Autodesk Fusion 360 part; units mm, degrees
(part 8 of 13)
  line L6244 (91.1132, -94.8176) -> (91.0017, -94.7608)
  line L6245 (101.955, -92.2213) -> (101.958, -92.1993)
  line L6246 (101.992, -92.133) -> (103.433, -90.6912)
  line L6247 (91.5604, -94.6723) -> (91.4719, -94.7608)
  line L6248 (103.086, -102.087) -> (103.021, -102.044)
  line L6249 (91.2368, -94.8372) -> (91.1132, -94.8176)
  line L6250 (103.457, -90.6736) -> (103.462, -90.6697)
  line L6251 (97.4257, -99.5716) -> (97.423, -99.5724)
  line L6252 (104.742, -90.9046) -> (103.574, -90.9046)
  line L6253 (105.254, -91.2108) -> (105.131, -91.2304)
  line L6254 (91.621, -94.5368) -> (91.6172, -94.5608)
  line L6255 (95.3324, -97.3037) -> (95.3333, -97.2973)
  line L6256 (95.7636, -96.8501) -> (95.7667, -96.8466)
  line L6257 (95.1296, -98.3423) -> (95.2181, -98.2538)
  line L6258 (95.6883, -98.2538) -> (95.7768, -98.3423)
  line L6259 (101.373, -94.0806) -> (101.373, -91.8718)
  line L6260 (103.434, -89.7635) -> (103.437, -89.76)
  line L6261 (95.2181, -98.901) -> (95.1296, -98.8125)
  line L6262 (95.8342, -96.8268) -> (96.127, -96.8268)
  line L6263 (108.504, -89.3456) -> (108.628, -89.4409)
  line L6264 (101.378, -91.8427) -> (101.379, -91.8363)
  line L6265 (95.2181, -98.2538) -> (95.3282, -98.1977)
  line L6266 (103.505, -89.7402) -> (107.62, -89.7402)
  line L6267 (107.684, -89.5652) -> (107.78, -89.4409)
  line L6268 (108.049, -89.2856) -> (108.204, -89.2652)
  line L6269 (95.7768, -98.3423) -> (95.8336, -98.4538)
  line L6270 (95.35, -97.2714) -> (95.3648, -97.2444)
  line L6271 (98.6272, -96.8268) -> (101.373, -94.0806)
  line L6272 (95.7694, -96.8458) -> (95.7746, -96.8419)
  line L6273 (95.8336, -98.4538) -> (95.8532, -98.5774)
  line L6274 (103.417, -89.7768) -> (103.434, -89.7635)
  line L6275 (105.131, -90.4304) -> (105.254, -90.45)
  line L6276 (96.127, -96.5818) -> (98.527, -96.5818)
  line L6277 (95.4532, -98.9774) -> (95.3296, -98.9578)
  line L6278 (105.007, -90.45) -> (105.131, -90.4304)
  line L6279 (95.7768, -98.8125) -> (95.6883, -98.901)
  line L6280 (108.204, -89.2652) -> (108.359, -89.2856)
  line L6281 (95.3311, -97.3062) -> (95.3324, -97.3037)
  line L6282 (101.373, -91.8718) -> (101.377, -91.8498)
  line L6283 (91.0017, -94.7608) -> (90.9132, -94.6723)
  line L6284 (92.1268, -99.3414) -> (97.3064, -99.3414)
  line L6285 (101.41, -91.7834) -> (103.417, -89.7768)
  line L6286 (95.6883, -98.901) -> (95.5768, -98.9578)
  line L6287 (95.0728, -98.4538) -> (95.1296, -98.3423)
  line L6288 (95.7458, -96.8634) -> (95.7636, -96.8501)
  line L6289 (95.3296, -98.9578) -> (95.2181, -98.901)
  line L6290 (95.3282, -97.3328) -> (95.3314, -97.3108)
  line L6291 (95.3648, -97.2444) -> (95.7458, -96.8634)
  line L6292 (95.5768, -98.9578) -> (95.4532, -98.9774)
  line L6293 (95.0532, -98.5774) -> (95.0728, -98.4538)
  line L6294 (107.904, -89.3456) -> (108.049, -89.2856)
  line L6295 (107.62, -89.7402) -> (107.624, -89.7099)
  line L6296 (103.475, -89.7489) -> (103.505, -89.7402)
  line L6297 (108.359, -89.2856) -> (108.504, -89.3456)
  line L6298 (107.624, -89.7099) -> (107.684, -89.5652)
  line L6299 (96.127, -96.8268) -> (96.127, -96.5818)
  line L6300 (101.377, -91.8498) -> (101.376, -91.8452)
  line L6301 (95.3333, -97.2973) -> (95.35, -97.2714)
  line L6302 (103.462, -90.6697) -> (103.492, -90.6633)
  line L6303 (95.8336, -98.701) -> (95.7768, -98.8125)
  line L6304 (103.445, -89.7553) -> (103.475, -89.7489)
  line L6305 (91.6172, -94.5608) -> (91.5604, -94.6723)
  line L6306 (95.1296, -98.8125) -> (95.0728, -98.701)
  line L6307 (98.527, -96.5818) -> (98.527, -96.8268)
  line L6308 (95.0728, -98.701) -> (95.0532, -98.5774)
  line L6309 (101.395, -91.8104) -> (101.41, -91.7834)
  line L6310 (103.437, -89.76) -> (103.44, -89.7592)
  line L6311 (95.8047, -96.8355) -> (95.8342, -96.8268)
  line L6312 (95.5782, -98.1977) -> (95.6883, -98.2538)
  line L6313 (95.3282, -98.1977) -> (95.3282, -97.3328)
  line L6314 (95.3314, -97.3108) -> (95.3311, -97.3062)
  line L6315 (101.379, -91.8363) -> (101.395, -91.8104)
  line L6316 (103.44, -89.7592) -> (103.445, -89.7553)
  line L6317 (95.7667, -96.8466) -> (95.7694, -96.8458)
  line L6318 (95.8532, -98.5774) -> (95.8336, -98.701)
  line L6319 (108.628, -89.4409) -> (108.724, -89.5652)
  line L6320 (122.123, -94.9134) -> (122, -94.8938)
  line L6321 (122.834, -95.4258) -> (122.812, -95.4226)
  line L6322 (121.743, -94.3898) -> (121.8, -94.2783)
  line L6323 (124.528, -95.406) -> (124.525, -95.4068)
  line L6324 (108.724, -90.1652) -> (108.628, -90.2895)
  line L6325 (98.7465, -97.057) -> (98.7438, -97.0578)
  line L6326 (122.773, -95.404) -> (122.746, -95.3892)
  line L6327 (101.619, -94.1615) -> (101.618, -94.1679)
  line L6328 (98.7496, -97.0535) -> (98.7465, -97.057)
  line L6329 (107.78, -90.2895) -> (107.684, -90.1652)
  line L6330 (98.527, -97.0768) -> (98.527, -97.3218)
  line L6331 (108.204, -90.4652) -> (108.049, -90.4448)
  line L6332 (96.127, -97.3218) -> (96.127, -97.0768)
  line L6333 (124.531, -95.4025) -> (124.528, -95.406)
  line L6334 (101.602, -94.1938) -> (101.587, -94.2208)
  line L6335 (95.7746, -96.8419) -> (95.8047, -96.8355)
  line L6336 (98.7085, -97.0681) -> (98.679, -97.0768)
  line L6337 (98.527, -97.3218) -> (96.127, -97.3218)
  line L6338 (101.587, -94.2208) -> (98.7674, -97.0402)
  line L6339 (124.52, -95.4107) -> (124.49, -95.4171)
  line L6340 (121.8, -94.2783) -> (121.888, -94.1898)
  line L6341 (121.743, -94.637) -> (121.723, -94.5134)
  line L6342 (107.624, -90.0205) -> (107.62, -89.9902)
  line L6343 (108.504, -90.3848) -> (108.359, -90.4448)
  line L6344 (95.5782, -97.3846) -> (95.5782, -98.1977)
  line L6345 (98.7438, -97.0578) -> (98.7386, -97.0617)
  line L6346 (108.784, -89.7099) -> (108.804, -89.8652)
  line L6347 (122.808, -95.4229) -> (122.805, -95.4216)
  line L6348 (101.621, -94.159) -> (101.619, -94.1615)
  line L6349 (98.679, -97.0768) -> (98.527, -97.0768)
  line L6350 (122.247, -94.8938) -> (122.123, -94.9134)
  line L6351 (98.527, -96.8268) -> (98.6272, -96.8268)
  line L6352 (121.888, -94.837) -> (121.8, -94.7485)
  line L6353 (107.78, -89.4409) -> (107.904, -89.3456)
  line L6354 (103.557, -89.9902) -> (101.623, -91.9236)
  line L6355 (101.623, -94.1324) -> (101.62, -94.1544)
  line L6356 (124.49, -95.4171) -> (124.46, -95.4258)
  line L6357 (122.746, -95.3892) -> (122.249, -94.8925)
  line L6358 (108.724, -89.5652) -> (108.784, -89.7099)
  line L6359 (122, -94.8938) -> (121.888, -94.837)
  line L6360 (121.8, -94.7485) -> (121.743, -94.637)
  line L6361 (108.804, -89.8652) -> (108.784, -90.0205)
  line L6362 (108.049, -90.4448) -> (107.904, -90.3848)
  line L6363 (101.376, -91.8452) -> (101.378, -91.8427)
  line L6364 (122.812, -95.4226) -> (122.808, -95.4229)
  line L6365 (122.249, -94.8925) -> (122.247, -94.8938)
  line L6366 (108.784, -90.0205) -> (108.724, -90.1652)
  line L6367 (101.62, -94.1544) -> (101.621, -94.159)
  line L6368 (107.684, -90.1652) -> (107.624, -90.0205)
  line L6369 (95.886, -97.0768) -> (95.5782, -97.3846)
  line L6370 (124.46, -95.4258) -> (122.834, -95.4258)
  line L6371 (107.904, -90.3848) -> (107.78, -90.2895)
  line L6372 (107.62, -89.9902) -> (103.557, -89.9902)
  line L6373 (108.359, -90.4448) -> (108.204, -90.4652)
  line L6374 (122.799, -95.4207) -> (122.773, -95.404)
  line L6375 (124.525, -95.4068) -> (124.52, -95.4107)
  line L6376 (98.7674, -97.0402) -> (98.7496, -97.0535)
  line L6377 (98.7386, -97.0617) -> (98.7085, -97.0681)
  line L6378 (101.618, -94.1679) -> (101.602, -94.1938)
  line L6379 (101.623, -91.9236) -> (101.623, -94.1324)
  line L6380 (108.628, -90.2895) -> (108.504, -90.3848)
  line L6381 (122.805, -95.4216) -> (122.799, -95.4207)
  line L6382 (121.723, -94.5134) -> (121.743, -94.3898)
  line L6383 (110.4, -92.9846) -> (110.305, -93.1089)
  line L6384 (122.504, -94.3898) -> (122.523, -94.5134)
  line L6385 (125.757, -92.0506) -> (124.484, -90.7776)
  line L6386 (113.296, -90.9442) -> (112.763, -91.4776)
  line L6387 (124.85, -94.7441) -> (124.874, -94.733)
  line L6388 (124.903, -94.7318) -> (125.692, -93.9424)
  line L6389 (122.447, -94.2783) -> (122.504, -94.3898)
  line L6390 (110.48, -92.6846) -> (110.46, -92.8399)
  line L6391 (124.778, -94.8048) -> (124.796, -94.7846)
  line L6392 (104.749, -96.9261) -> (104.816, -97.0341)
  line L6393 (122.451, -94.7405) -> (122.886, -95.1758)
  line L6394 (112.734, -91.4991) -> (112.704, -91.5055)
  line L6395 (121.888, -94.1898) -> (122, -94.133)
  line L6396 (109.297, -92.8096) -> (108.865, -92.8096)
  line L6397 (110.46, -92.8399) -> (110.4, -92.9846)
  line L6398 (124.408, -95.1758) -> (124.499, -95.0854)
  line L6399 (113.296, -90.9442) -> (113.296, -90.9442)
  line L6400 (113.463, -90.7776) -> (113.296, -90.9442)
  line L6401 (125.757, -93.8774) -> (125.757, -92.0506)
  line L6402 (125.692, -93.9424) -> (125.757, -93.8774)
  line L6403 (124.874, -94.733) -> (124.883, -94.7343)
  line L6404 (109.456, -93.1089) -> (109.361, -92.9846)
  line L6405 (104.715, -97.8403) -> (104.593, -97.9556)
  line L6406 (124.824, -94.7516) -> (124.85, -94.7441)
  line L6407 (110.4, -92.3846) -> (110.46, -92.5293)
  line L6408 (109.301, -92.8399) -> (109.297, -92.8096)
  line L6409 (104.89, -97.3791) -> (104.866, -97.5447)
  line L6410 (122.358, -94.1898) -> (122.447, -94.2783)
  line L6411 (112.742, -91.4944) -> (112.739, -91.4952)
  line L6412 (122.123, -94.1134) -> (122.247, -94.133)
  line L6413 (109.361, -92.9846) -> (109.301, -92.8399)
  line L6414 (104.866, -97.5447) -> (104.807, -97.701)
  line L6415 (110.305, -93.1089) -> (110.18, -93.2042)
  line L6416 (112.745, -91.4909) -> (112.742, -91.4944)
  line L6417 (104.807, -97.701) -> (104.715, -97.8403)
  line L6418 (124.892, -94.7318) -> (124.903, -94.7318)
  line L6419 (122.523, -94.5134) -> (122.504, -94.637)
  line L6420 (104.593, -97.9556) -> (104.45, -98.0412)
  line L6421 (124.81, -94.7622) -> (124.818, -94.7584)
  line L6422 (124.484, -90.7776) -> (113.463, -90.7776)
  line L6423 (124.796, -94.7846) -> (124.81, -94.7622)
  line L6424 (124.883, -94.7343) -> (124.892, -94.7318)
  line L6425 (104.816, -97.0341) -> (104.871, -97.192)
  line L6426 (124.778, -94.8061) -> (124.778, -94.8048)
  line L6427 (104.45, -98.0412) -> (104.291, -98.0929)
  line L6428 (112.704, -91.5055) -> (112.674, -91.5142)
  line L6429 (122, -94.133) -> (122.123, -94.1134)
  line L6430 (96.127, -97.0768) -> (95.886, -97.0768)
  line L6431 (112.763, -91.4776) -> (112.745, -91.4909)
  line L6432 (125.692, -93.9424) -> (125.692, -93.9424)
  line L6433 (108.865, -92.8096) -> (104.749, -96.9261)
  line L6434 (124.499, -95.0854) -> (124.778, -94.8061)
  line L6435 (110.18, -93.2042) -> (110.036, -93.2642)
  line L6436 (111.228, -91.5142) -> (110.381, -92.3604)
  line L6437 (109.725, -93.2642) -> (109.58, -93.2042)
  line L6438 (110.381, -92.3604) -> (110.4, -92.3846)
  line L6439 (112.739, -91.4952) -> (112.734, -91.4991)
  line L6440 (122.886, -95.1758) -> (124.408, -95.1758)
  line L6441 (112.674, -91.5142) -> (111.228, -91.5142)
  line L6442 (110.46, -92.5293) -> (110.48, -92.6846)
  line L6443 (124.818, -94.7584) -> (124.824, -94.7516)
  line L6444 (122.504, -94.637) -> (122.451, -94.7405)
  line L6445 (122.247, -94.133) -> (122.358, -94.1898)
  line L6446 (109.58, -93.2042) -> (109.456, -93.1089)
  line L6447 (104.311, -96.628) -> (104.469, -96.6841)
  line L6448 (109.725, -92.105) -> (109.88, -92.0846)
  line L6449 (103.678, -96.7672) -> (103.821, -96.6796)
  line L6450 (103.468, -97.0247) -> (103.559, -96.8842)
  line L6451 (111.116, -91.2793) -> (111.146, -91.2729)
  line L6452 (108.746, -92.5794) -> (108.749, -92.5786)
  line L6453 (103.406, -97.5141) -> (103.39, -97.3477)
  line L6454 (108.749, -92.5786) -> (108.754, -92.5747)
  line L6455 (109.297, -92.5596) -> (109.301, -92.5293)
  line L6456 (104.572, -96.7495) -> (108.725, -92.5962)
  line L6457 (113.343, -90.5474) -> (113.346, -90.5466)
  line L6458 (113.381, -90.5363) -> (113.411, -90.5276)
  line L6459 (124.536, -90.5276) -> (124.558, -90.5308)
  line L6460 (104.124, -98.108) -> (103.959, -98.0859)
  line L6461 (104.145, -96.6082) -> (104.311, -96.628)
  line L6462 (104.871, -97.192) -> (104.89, -97.3582)
  line L6463 (110.205, -92.1836) -> (111.087, -91.3008)
  line L6464 (124.625, -90.5642) -> (125.971, -91.9104)
  line L6465 (109.361, -92.3846) -> (109.456, -92.2603)
  line L6466 (113.323, -90.5642) -> (113.34, -90.5509)
  line L6467 (124.558, -90.5308) -> (124.563, -90.5305)
  line L6468 (109.88, -92.0846) -> (110.036, -92.105)
  line L6469 (103.959, -98.0859) -> (103.802, -98.0276)
  line L6470 (111.146, -91.2729) -> (111.176, -91.2642)
  line L6471 (113.351, -90.5427) -> (113.381, -90.5363)
  line L6472 (103.459, -97.6728) -> (103.406, -97.5141)
  line L6473 (103.411, -97.1818) -> (103.468, -97.0247)
  line L6474 (109.58, -92.165) -> (109.725, -92.105)
  line L6475 (113.34, -90.5509) -> (113.343, -90.5474)
  line L6476 (104.469, -96.6841) -> (104.572, -96.7495)
  line L6477 (104.291, -98.0929) -> (104.124, -98.108)
  line L6478 (110.036, -93.2642) -> (109.88, -93.2846)
  line L6479 (108.725, -92.5962) -> (108.743, -92.5829)
  line L6480 (108.743, -92.5829) -> (108.746, -92.5794)
  line L6481 (109.456, -92.2603) -> (109.58, -92.165)
  line L6482 (103.559, -96.8842) -> (103.678, -96.7672)
  line L6483 (103.39, -97.3477) -> (103.411, -97.1818)
  line L6484 (125.988, -91.9313) -> (125.988, -91.934)
  line L6485 (108.754, -92.5747) -> (108.784, -92.5683)
  line L6486 (108.814, -92.5596) -> (109.297, -92.5596)
  line L6487 (111.087, -91.3008) -> (111.105, -91.2875)
  line L6488 (125.984, -91.9282) -> (125.988, -91.9313)
  line L6489 (103.979, -96.6257) -> (104.145, -96.6082)
  line L6490 (103.662, -97.9361) -> (103.546, -97.8158)
  line L6491 (103.802, -98.0276) -> (103.662, -97.9361)
  line L6492 (113.346, -90.5466) -> (113.351, -90.5427)
  line L6493 (109.88, -93.2846) -> (109.725, -93.2642)
  line L6494 (103.821, -96.6796) -> (103.979, -96.6257)
  line L6495 (124.598, -90.5494) -> (124.625, -90.5642)
  line L6496 (113.119, -90.7674) -> (113.323, -90.5642)
  line L6497 (125.988, -91.934) -> (125.992, -91.9392)
  line L6498 (111.111, -91.2832) -> (111.116, -91.2793)
  line L6499 (124.565, -90.5318) -> (124.572, -90.5327)
  line L6500 (111.176, -91.2642) -> (112.623, -91.2642)
  line L6501 (110.036, -92.105) -> (110.18, -92.165)
  line L6502 (125.971, -91.9104) -> (125.984, -91.9282)
  line L6503 (124.563, -90.5305) -> (124.565, -90.5318)
  line L6504 (104.89, -97.3582) -> (104.89, -97.3791)
  line L6505 (103.546, -97.8158) -> (103.459, -97.6728)
  line L6506 (124.572, -90.5327) -> (124.598, -90.5494)
  line L6507 (112.623, -91.2642) -> (113.119, -90.7674)
  line L6508 (109.301, -92.5293) -> (109.361, -92.3846)
  line L6509 (108.784, -92.5683) -> (108.814, -92.5596)
  line L6510 (113.411, -90.5276) -> (124.536, -90.5276)
  line L6511 (111.266, -90.1652) -> (111.206, -90.0205)
  line L6512 (125.971, -94.0176) -> (125.869, -94.1192)
  line L6513 (125.022, -94.962) -> (125.02, -94.9628)
  line L6514 (125.869, -94.1192) -> (125.869, -94.1192)
  line L6515 (111.266, -89.5652) -> (111.284, -89.541)
  line L6516 (111.941, -89.2856) -> (112.085, -89.3456)
  line L6517 (112.365, -89.7099) -> (112.385, -89.8652)
  line L6518 (112.085, -90.3848) -> (111.941, -90.4448)
  line L6519 (111.108, -91.284) -> (111.111, -91.2832)
  line L6520 (113.119, -90.7674) -> (113.119, -90.7674)
  line L6521 (110.18, -92.165) -> (110.205, -92.1836)
  line L6522 (125.999, -91.9693) -> (126.007, -91.9988)
  line L6523 (125.992, -91.9392) -> (125.999, -91.9693)
  line L6524 (125.869, -94.1192) -> (125.043, -94.9452)
  line L6525 (111.206, -90.0205) -> (111.185, -89.8652)
  line L6526 (111.284, -89.541) -> (110.692, -88.9488)
  line L6527 (110.78, -88.7039) -> (110.805, -88.7206)
  line L6528 (110.773, -88.703) -> (110.78, -88.7039)
  line L6529 (94.6272, -97.0402) -> (94.627, -97.0403)
  line L6530 (111.485, -90.3848) -> (111.361, -90.2895)
  line L6531 (95.8017, -95.8443) -> (95.785, -95.8702)
  line L6532 (111.361, -90.2895) -> (111.266, -90.1652)
  line L6533 (112.085, -89.3456) -> (112.21, -89.4409)
  line L6534 (125.025, -94.9585) -> (125.022, -94.962)
  line L6535 (110.692, -88.9488) -> (97.7656, -88.9488)
  line L6536 (95.8068, -95.8088) -> (95.8036, -95.8308)
  line L6537 (111.785, -90.4652) -> (111.63, -90.4448)
  line L6538 (110.832, -88.7354) -> (111.461, -89.3642)
  line L6539 (125.043, -94.9452) -> (125.025, -94.9585)
  line L6540 (111.485, -89.3456) -> (111.63, -89.2856)
  line L6541 (124.984, -94.9731) -> (124.956, -94.9814)
  line L6542 (124.956, -94.9814) -> (124.548, -95.3892)
  line L6543 (125.986, -93.9906) -> (125.971, -94.0176)
  line L6544 (126.003, -93.9583) -> (126.002, -93.9647)
  line L6545 (111.461, -89.3642) -> (111.485, -89.3456)
  line L6546 (126.002, -93.9647) -> (125.986, -93.9906)
  line L6547 (124.548, -95.3892) -> (124.531, -95.4025)
  line L6548 (111.63, -89.2856) -> (111.785, -89.2652)
  line L6549 (126.005, -93.9558) -> (126.003, -93.9583)
  line L6550 (112.305, -89.5652) -> (112.365, -89.7099)
  line L6551 (110.805, -88.7206) -> (110.832, -88.7354)
  line L6552 (111.185, -89.8652) -> (111.206, -89.7099)
  line L6553 (112.385, -89.8652) -> (112.365, -90.0205)
  line L6554 (97.7656, -88.9488) -> (95.8068, -90.9076)
  line L6555 (125.014, -94.9667) -> (124.984, -94.9731)
  line L6556 (111.63, -90.4448) -> (111.485, -90.3848)
  line L6557 (125.02, -94.9628) -> (125.014, -94.9667)
  line L6558 (126.004, -93.9512) -> (126.005, -93.9558)
  line L6559 (111.785, -89.2652) -> (111.941, -89.2856)
  line L6560 (126.007, -91.9988) -> (126.007, -93.9292)
  line L6561 (110.766, -88.702) -> (110.771, -88.7017)
  line L6562 (110.771, -88.7017) -> (110.773, -88.703)
  line L6563 (111.105, -91.2875) -> (111.108, -91.284)
  line L6564 (95.8026, -95.8379) -> (95.8017, -95.8443)
  line L6565 (95.8039, -95.8354) -> (95.8026, -95.8379)
  line L6566 (111.941, -90.4448) -> (111.785, -90.4652)
  line L6567 (126.007, -93.9292) -> (126.004, -93.9512)
  line L6568 (112.21, -90.2895) -> (112.085, -90.3848)
  line L6569 (112.21, -89.4409) -> (112.305, -89.5652)
  line L6570 (95.8068, -90.9076) -> (95.8068, -95.8088)
  line L6571 (112.305, -90.1652) -> (112.21, -90.2895)
  line L6572 (95.8036, -95.8308) -> (95.8039, -95.8354)
  line L6573 (111.206, -89.7099) -> (111.266, -89.5652)
  line L6574 (95.785, -95.8702) -> (95.7702, -95.8972)
  line L6575 (118.156, -93.4328) -> (118.011, -93.4928)
  line L6576 (95.5786, -90.7944) -> (95.5934, -90.7674)
  line L6577 (91.6172, -97.2346) -> (91.6368, -97.3582)
  line L6578 (110.744, -88.6988) -> (110.766, -88.702)
  line L6579 (90.8564, -97.4818) -> (90.8368, -97.3582)
  line L6580 (118.436, -93.0685) -> (118.376, -93.2132)
  line L6581 (95.5568, -95.757) -> (95.5568, -90.8558)
  line L6582 (97.649, -88.7178) -> (97.6542, -88.7139)
  line L6583 (97.6843, -88.7075) -> (97.7138, -88.6988)
  line L6584 (118.376, -93.2132) -> (118.28, -93.3375)
  line L6585 (91.5604, -97.5933) -> (91.4719, -97.6818)
  line L6586 (118.156, -92.3936) -> (118.28, -92.4889)
  line L6587 (92.227, -96.5818) -> (94.627, -96.5818)
  line L6588 (94.627, -97.0403) -> (94.627, -97.3218)
  line L6589 (90.8368, -97.3582) -> (90.8564, -97.2346)
  line L6590 (118.436, -92.7579) -> (118.456, -92.9132)
  line L6591 (91.695, -97.0768) -> (91.5902, -97.1816)
  line L6592 (91.5784, -96.8458) -> (91.5836, -96.8419)
  line L6593 (112.365, -90.0205) -> (112.305, -90.1652)
  line L6594 (91.3604, -97.7386) -> (91.2368, -97.7582)
  line L6595 (91.6172, -97.4818) -> (91.5604, -97.5933)
  line L6596 (91.0017, -97.0346) -> (91.1132, -96.9778)
  line L6597 (90.9132, -97.1231) -> (91.0017, -97.0346)
  line L6598 (91.1132, -97.7386) -> (91.0017, -97.6818)
  line L6599 (94.627, -97.3218) -> (92.227, -97.3218)
  line L6600 (91.4134, -97.0048) -> (91.5548, -96.8634)
  line L6601 (90.8564, -97.2346) -> (90.9132, -97.1231)
  line L6602 (95.7702, -95.8972) -> (94.6272, -97.0402)
  line L6603 (94.627, -96.6868) -> (95.5568, -95.757)
  line L6604 (91.1132, -96.9778) -> (91.2368, -96.9582)
  line L6605 (92.227, -96.8268) -> (92.227, -96.5818)
  line L6606 (90.9132, -97.5933) -> (90.8564, -97.4818)
  line L6607 (97.6254, -88.7354) -> (97.6432, -88.7221)
  line L6608 (97.6463, -88.7186) -> (97.649, -88.7178)
  line L6609 (118.456, -92.9132) -> (118.436, -93.0685)
  line L6610 (97.6432, -88.7221) -> (97.6463, -88.7186)
  line L6611 (91.4719, -97.6818) -> (91.3604, -97.7386)
  line L6612 (91.2368, -96.9582) -> (91.3604, -96.9778)
  line L6613 (91.5757, -96.8466) -> (91.5784, -96.8458)
  line L6614 (95.56, -90.8338) -> (95.5597, -90.8292)
  line L6615 (118.28, -93.3375) -> (118.156, -93.4328)
  line L6616 (95.5934, -90.7674) -> (97.6254, -88.7354)
  line L6617 (95.5568, -90.8558) -> (95.56, -90.8338)
  line L6618 (91.6137, -96.8355) -> (91.6432, -96.8268)
  line L6619 (95.5619, -90.8203) -> (95.5786, -90.7944)
  line L6620 (91.5836, -96.8419) -> (91.6137, -96.8355)
  line L6621 (91.2368, -97.7582) -> (91.1132, -97.7386)
  line L6622 (91.0017, -97.6818) -> (90.9132, -97.5933)
  line L6623 (91.5548, -96.8634) -> (91.5726, -96.8501)
  line L6624 (91.6432, -96.8268) -> (92.227, -96.8268)
  line L6625 (92.227, -97.0768) -> (91.695, -97.0768)
  line L6626 (118.28, -92.4889) -> (118.376, -92.6132)
  line L6627 (91.6368, -97.3582) -> (91.6172, -97.4818)
  line L6628 (91.5726, -96.8501) -> (91.5757, -96.8466)
  line L6629 (91.5902, -97.1816) -> (91.6172, -97.2346)
  line L6630 (118.011, -92.3336) -> (118.156, -92.3936)
  line L6631 (118.376, -92.6132) -> (118.436, -92.7579)
  line L6632 (92.227, -97.3218) -> (92.227, -97.0768)
  line L6633 (95.5597, -90.8292) -> (95.561, -90.8267)
  line L6634 (97.6542, -88.7139) -> (97.6843, -88.7075)
  line L6635 (94.627, -96.5818) -> (94.627, -96.6868)
  line L6636 (97.7138, -88.6988) -> (110.744, -88.6988)
  line L6637 (91.3604, -96.9778) -> (91.4134, -97.0048)
  line L6638 (95.561, -90.8267) -> (95.5619, -90.8203)
  line L6639 (117.295, -93.6508) -> (117.295, -95.7843)
  line L6640 (117.295, -95.7843) -> (117.341, -95.7898)
  line L6641 (117.048, -93.5724) -> (117.049, -93.5699)
  line L6642 (117.837, -96.8628) -> (117.745, -97.0021)
  line L6643 (114.566, -92.3338) -> (114.626, -92.4785)
  line L6644 (117.082, -93.5106) -> (117.355, -93.2374)
  line L6645 (114.346, -93.1534) -> (114.201, -93.2134)
  line L6646 (117.624, -97.1174) -> (117.48, -97.203)
  line L6647 (117.701, -93.4928) -> (117.556, -93.4328)
  line L6648 (116.708, -95.929) -> (116.851, -95.8414)
  line L6649 (117.432, -92.4889) -> (117.556, -92.3936)
  line L6650 (114.646, -92.6338) -> (114.626, -92.7891)
  line L6651 (116.489, -96.8346) -> (116.437, -96.6759)
  line L6652 (114.201, -93.2134) -> (114.046, -93.2338)
  line L6653 (117.045, -93.599) -> (117.048, -93.577)
  line L6654 (117.048, -93.577) -> (117.048, -93.5724)
  line L6655 (117.92, -96.52) -> (117.92, -96.5409)
  line L6656 (117.321, -97.2547) -> (117.154, -97.2698)
  line L6657 (116.437, -96.6759) -> (116.42, -96.5095)
  line L6658 (116.692, -97.0979) -> (116.576, -96.9776)
  line L6659 (117.05, -93.5635) -> (117.067, -93.5376)
  line L6660 (117.276, -93.0685) -> (117.256, -92.9132)
  line L6661 (116.989, -97.2477) -> (116.832, -97.1894)
  line L6662 (114.47, -93.0581) -> (114.346, -93.1534)
  line L6663 (118.011, -93.4928) -> (117.856, -93.5132)
  line L6664 (117.856, -92.3132) -> (118.011, -92.3336)
  line L6665 (116.589, -96.046) -> (116.708, -95.929)
  line L6666 (117.902, -96.3538) -> (117.92, -96.52)
  line L6667 (116.576, -96.9776) -> (116.489, -96.8346)
  line L6668 (117.897, -96.7065) -> (117.837, -96.8628)
  line L6669 (114.566, -92.9338) -> (114.47, -93.0581)
  line L6670 (117.049, -93.5699) -> (117.05, -93.5635)
  line L6671 (117.532, -93.4142) -> (117.295, -93.6508)
  line L6672 (117.745, -97.0021) -> (117.624, -97.1174)
  line L6673 (117.48, -97.203) -> (117.321, -97.2547)
  line L6674 (117.154, -97.2698) -> (116.989, -97.2477)
  line L6675 (116.851, -95.8414) -> (117.009, -95.7875)
  line L6676 (117.256, -92.9132) -> (117.276, -92.7579)
  line L6677 (117.276, -92.7579) -> (117.336, -92.6132)
  line L6678 (114.346, -92.1142) -> (114.47, -92.2095)
  line L6679 (117.556, -93.4328) -> (117.532, -93.4142)
  line L6680 (117.758, -96.0541) -> (117.847, -96.1959)
  line L6681 (117.701, -92.3336) -> (117.856, -92.3132)
  line L6682 (114.626, -92.4785) -> (114.646, -92.6338)
  line L6683 (116.832, -97.1894) -> (116.692, -97.0979)
  line L6684 (116.498, -96.1865) -> (116.589, -96.046)
  line L6685 (117.045, -95.7837) -> (117.045, -93.599)
  line L6686 (116.42, -96.5095) -> (116.441, -96.3436)
  line L6687 (117.009, -95.7875) -> (117.045, -95.7837)
  line L6688 (117.92, -96.5409) -> (117.897, -96.7065)
  line L6689 (117.847, -96.1959) -> (117.902, -96.3538)
  line L6690 (117.336, -92.6132) -> (117.432, -92.4889)
  line L6691 (114.626, -92.7891) -> (114.566, -92.9338)
  line L6692 (114.47, -92.2095) -> (114.566, -92.3338)
  line L6693 (117.355, -93.2374) -> (117.336, -93.2132)
  line L6694 (117.556, -92.3936) -> (117.701, -92.3336)
  line L6695 (114.201, -92.0542) -> (114.346, -92.1142)
  line L6696 (117.64, -95.9355) -> (117.758, -96.0541)
  line L6697 (117.336, -93.2132) -> (117.276, -93.0685)
  line L6698 (117.341, -95.7898) -> (117.499, -95.8459)
  line L6699 (117.856, -93.5132) -> (117.701, -93.4928)
  line L6700 (117.499, -95.8459) -> (117.64, -95.9355)
  line L6701 (116.441, -96.3436) -> (116.498, -96.1865)
  line L6702 (117.067, -93.5376) -> (117.082, -93.5106)
  line L6703 (124.375, -94.6186) -> (124.372, -94.6194)
  line L6704 (113.746, -92.1142) -> (113.891, -92.0542)
  line L6705 (114.396, -96.8628) -> (114.303, -97.0021)
  line L6706 (113.879, -97.2547) -> (113.713, -97.2698)
  line L6707 (113.25, -97.0979) -> (113.134, -96.9776)
  line L6708 (124.344, -91.2098) -> (124.371, -91.2246)
  line L6709 (114.455, -96.7065) -> (114.396, -96.8628)
  line L6710 (124.372, -94.6194) -> (124.367, -94.6233)
  line L6711 (125.425, -92.2838) -> (125.429, -92.2869)
  line L6712 (125.449, -92.3544) -> (125.449, -93.4974)
  line L6713 (113.547, -97.2477) -> (113.39, -97.1894)
  line L6714 (125.433, -92.2948) -> (125.44, -92.3249)
  line L6715 (125.44, -92.3249) -> (125.449, -92.3544)
  line L6716 (125.445, -93.5194) -> (125.446, -93.524)
  line L6717 (112.979, -96.5095) -> (113, -96.3436)
  line L6718 (113.39, -97.1894) -> (113.25, -97.0979)
  line L6719 (124.367, -94.6233) -> (124.337, -94.6297)
  line L6720 (113.853, -93.1979) -> (113.853, -95.7843)
  line L6721 (113.147, -96.046) -> (113.267, -95.929)
  line L6722 (112.995, -96.6759) -> (112.979, -96.5095)
  line L6723 (125.446, -93.524) -> (125.444, -93.5265)
  line L6724 (125.412, -92.266) -> (125.425, -92.2838)
  line L6725 (113.048, -96.8346) -> (112.995, -96.6759)
  line L6726 (114.316, -96.0541) -> (114.405, -96.1959)
  line L6727 (114.057, -95.8459) -> (114.198, -95.9355)
  line L6728 (113.446, -92.6338) -> (113.466, -92.4785)
  line L6729 (113.466, -92.7891) -> (113.446, -92.6338)
  line L6730 (124.318, -91.1931) -> (124.344, -91.2098)
  line L6731 (124.311, -91.1922) -> (124.318, -91.1931)
  line L6732 (125.429, -92.2869) -> (125.43, -92.2896)
  line L6733 (114.478, -96.5409) -> (114.455, -96.7065)
  line L6734 (114.303, -97.0021) -> (114.182, -97.1174)
  line L6735 (113.9, -95.7898) -> (114.057, -95.8459)
  line L6736 (113.409, -95.8414) -> (113.567, -95.7875)
  line L6737 (113, -96.3436) -> (113.057, -96.1865)
  line L6738 (114.038, -97.203) -> (113.879, -97.2547)
  line L6739 (114.46, -96.3538) -> (114.478, -96.52)
  line L6740 (113.134, -96.9776) -> (113.048, -96.8346)
  line L6741 (113.891, -93.2134) -> (113.853, -93.1979)
  line L6742 (114.198, -95.9355) -> (114.316, -96.0541)
  line L6743 (114.405, -96.1959) -> (114.46, -96.3538)
  line L6744 (113.713, -97.2698) -> (113.547, -97.2477)
  line L6745 (125.449, -93.4974) -> (125.445, -93.5194)
  line L6746 (125.43, -92.2896) -> (125.433, -92.2948)
  line L6747 (124.396, -94.6018) -> (124.378, -94.6151)
  line L6748 (125.444, -93.5265) -> (125.443, -93.5329)
  line L6749 (114.182, -97.1174) -> (114.038, -97.203)
  line L6750 (113.526, -92.9338) -> (113.466, -92.7891)
  line L6751 (113.267, -95.929) -> (113.409, -95.8414)
  line L6752 (125.412, -93.5858) -> (124.396, -94.6018)
  line L6753 (113.603, -95.7837) -> (113.603, -93.0343)
  line L6754 (124.371, -91.2246) -> (125.412, -92.266)
  line L6755 (124.304, -91.1912) -> (124.309, -91.1909)
  line L6756 (113.567, -95.7875) -> (113.603, -95.7837)
  line L6757 (114.046, -92.0338) -> (114.201, -92.0542)
  line L6758 (125.427, -93.5588) -> (125.412, -93.5858)
  line L6759 (124.378, -94.6151) -> (124.375, -94.6186)
  line L6760 (113.853, -95.7843) -> (113.9, -95.7898)
  line L6761 (113.603, -93.0343) -> (113.526, -92.9338)
  line L6762 (113.057, -96.1865) -> (113.147, -96.046)
  line L6763 (113.891, -92.0542) -> (114.046, -92.0338)
  line L6764 (113.622, -92.2095) -> (113.746, -92.1142)
  line L6765 (114.046, -93.2338) -> (113.891, -93.2134)
  line L6766 (114.478, -96.52) -> (114.478, -96.5409)
  line L6767 (113.526, -92.3338) -> (113.622, -92.2095)
  line L6768 (124.23, -91.438) -> (113.488, -91.438)
  line L6769 (125.199, -93.4456) -> (125.199, -92.4062)
  line L6770 (112.559, -92.41) -> (112.619, -92.5547)
  line L6771 (123.578, -94.7485) -> (123.521, -94.637)
  line L6772 (125.443, -93.5329) -> (125.427, -93.5588)
  line L6773 (124.309, -91.1909) -> (124.311, -91.1922)
  line L6774 (125.199, -92.4062) -> (124.23, -91.438)
  line L6775 (112.54, -92.3858) -> (112.559, -92.41)
  line L6776 (112.639, -92.71) -> (112.619, -92.8653)
  line L6777 (112.619, -92.8653) -> (112.559, -93.01)
  line L6778 (113.466, -92.4785) -> (113.526, -92.3338)
  line L6779 (100.591, -89.5793) -> (100.679, -89.4908)
  line L6780 (98.9243, -91.977) -> (98.9216, -91.9778)
  line L6781 (112.468, -85.2378) -> (112.324, -85.1778)
  line L6782 (100.738, -90.1678) -> (98.9452, -91.9602)
  line L6783 (112.044, -84.8135) -> (112.024, -84.6582)
  line L6784 (90.7548, -91.97) -> (90.7352, -91.8464)
  line L6785 (91.0116, -91.466) -> (91.1352, -91.4464)
  line L6786 (101.185, -83.5831) -> (101.215, -83.5767)
  line L6787 (101.18, -83.587) -> (101.185, -83.5831)
  line L6788 (100.679, -89.4908) -> (100.791, -89.434)
  line L6789 (93.3062, -91.4813) -> (93.3071, -91.4749)
  line L6790 (100.791, -89.434) -> (100.914, -89.4144)
  line L6791 (113.048, -85.0825) -> (112.924, -85.1778)
  line L6792 (113.143, -84.9582) -> (113.048, -85.0825)
  line L6793 (98.8568, -91.9968) -> (98.527, -91.9968)
  line L6794 (111.658, -83.568) -> (111.68, -83.5712)
  line L6795 (113.224, -84.6582) -> (113.203, -84.8135)
  line L6796 (91.1352, -91.4464) -> (91.2588, -91.466)
  line L6797 (93.3238, -91.449) -> (93.3386, -91.422)
  line L6798 (91.4588, -91.6113) -> (91.5156, -91.7228)
  line L6799 (113.203, -84.5029) -> (113.224, -84.6582)
  line L6800 (93.6124, -91.5018) -> (94.627, -91.5018)
  line L6801 (113.048, -84.2339) -> (113.143, -84.3582)
  line L6802 (113.143, -84.3582) -> (113.203, -84.5029)
  line L6803 (90.7352, -91.8464) -> (90.7548, -91.7228)
  line L6804 (93.3386, -91.422) -> (101.156, -83.6046)
  line L6805 (112.123, -84.334) -> (111.607, -83.818)
  line L6806 (91.5194, -91.7468) -> (92.227, -91.7468)
  line L6807 (93.3052, -91.4884) -> (93.3049, -91.4838)
  line L6808 (90.9001, -92.17) -> (90.8116, -92.0815)
  line L6809 (91.0116, -92.2268) -> (90.9001, -92.17)
  line L6810 (111.607, -83.818) -> (101.296, -83.818)
  line L6811 (92.227, -91.7468) -> (92.227, -91.5018)
  line L6812 (101.177, -83.5878) -> (101.18, -83.587)
  line L6813 (90.9001, -91.5228) -> (91.0116, -91.466)
  line L6814 (93.3071, -91.4749) -> (93.3238, -91.449)
  line L6815 (94.627, -91.5018) -> (94.627, -92.2418)
  line L6816 (91.1352, -92.2464) -> (91.0116, -92.2268)
  line L6817 (112.044, -84.5029) -> (112.104, -84.3582)
  line L6818 (90.7548, -91.7228) -> (90.8116, -91.6113)
  line L6819 (101.238, -89.5793) -> (101.295, -89.6908)
  line L6820 (96.127, -91.5018) -> (98.527, -91.5018)
  line L6821 (90.8116, -91.6113) -> (90.9001, -91.5228)
  line L6822 (112.024, -84.6582) -> (112.044, -84.5029)
  line L6823 (90.8116, -92.0815) -> (90.7548, -91.97)
  line L6824 (113.203, -84.8135) -> (113.143, -84.9582)
  line L6825 (112.199, -85.0825) -> (112.104, -84.9582)
  line L6826 (112.624, -85.2582) -> (112.468, -85.2378)
  line L6827 (91.2588, -91.466) -> (91.3703, -91.5228)
  line L6828 (93.3032, -91.5018) -> (93.3052, -91.4884)
  line L6829 (101.174, -83.5913) -> (101.177, -83.5878)
  line L6830 (92.227, -91.5018) -> (93.3032, -91.5018)
  line L6831 (101.296, -83.818) -> (93.6124, -91.5018)
  line L6832 (112.779, -85.2378) -> (112.624, -85.2582)
  line L6833 (91.3703, -91.5228) -> (91.4588, -91.6113)
  line L6834 (101.156, -83.6046) -> (101.174, -83.5913)
  line L6835 (101.244, -83.568) -> (111.658, -83.568)
  line L6836 (93.3049, -91.4838) -> (93.3062, -91.4813)
  line L6837 (101.215, -83.5767) -> (101.244, -83.568)
  line L6838 (101.038, -89.434) -> (101.149, -89.4908)
  line L6839 (91.5156, -91.7228) -> (91.5194, -91.7468)
  line L6840 (100.534, -89.6908) -> (100.591, -89.5793)
  line L6841 (92.227, -92.2418) -> (92.227, -91.9968)
  line L6842 (98.527, -92.2418) -> (96.127, -92.2418)
  line L6843 (100.534, -89.938) -> (100.514, -89.8144)
  line L6844 (101.149, -90.138) -> (101.038, -90.1948)
  line L6845 (101.038, -90.1948) -> (100.914, -90.2144)
  line L6846 (98.9274, -91.9735) -> (98.9243, -91.977)
  line L6847 (100.561, -89.991) -> (100.534, -89.938)
  line L6848 (101.238, -90.0495) -> (101.149, -90.138)
  line L6849 (101.314, -89.8144) -> (101.295, -89.938)
  line L6850 (98.9164, -91.9817) -> (98.8863, -91.9881)
  line L6851 (98.527, -91.9968) -> (98.527, -92.2418)
  line L6852 (96.127, -92.2418) -> (96.127, -91.5018)
  line L6853 (100.514, -89.8144) -> (100.534, -89.6908)
  line L6854 (98.527, -91.7468) -> (98.805, -91.7468)
  line L6855 (98.527, -91.5018) -> (98.527, -91.7468)
  line L6856 (100.791, -90.1948) -> (100.738, -90.1678)
  line L6857 (100.914, -90.2144) -> (100.791, -90.1948)
  line L6858 (101.295, -89.938) -> (101.238, -90.0495)
  line L6859 (101.149, -89.4908) -> (101.238, -89.5793)
  line L6860 (129.766, -91.8672) -> (129.621, -91.8072)
  line L6861 (101.295, -89.6908) -> (101.314, -89.8144)
  line L6862 (129.921, -91.8876) -> (129.766, -91.8672)
  line L6863 (98.9216, -91.9778) -> (98.9164, -91.9817)
  line L6864 (98.9452, -91.9602) -> (98.9274, -91.9735)
  line L6865 (98.8863, -91.9881) -> (98.8568, -91.9968)
  line L6866 (98.805, -91.7468) -> (100.561, -89.991)
  line L6867 (130.076, -91.8672) -> (129.921, -91.8876)
  line L6868 (129.497, -91.7119) -> (129.401, -91.5876)
  line L6869 (129.401, -91.5876) -> (129.341, -91.4429)
  line L6870 (129.621, -90.768) -> (129.766, -90.708)
  line L6871 (135.943, -71.3229) -> (136.061, -71.4415)
  line L6872 (136.061, -71.4415) -> (136.15, -71.5833)
  line L6873 (129.341, -91.4429) -> (129.321, -91.2876)
  line L6874 (130.441, -90.9876) -> (130.501, -91.1323)
  line L6875 (130.221, -90.768) -> (130.345, -90.8633)
  line L6876 (130.521, -91.2876) -> (130.501, -91.4429)
  line L6877 (100.914, -89.4144) -> (101.038, -89.434)
  line L6878 (136.205, -71.7412) -> (136.223, -71.9074)
  line L6879 (136.15, -71.5833) -> (136.205, -71.7412)
  line L6880 (130.345, -90.8633) -> (130.441, -90.9876)
  line L6881 (136.223, -71.9074) -> (136.223, -71.9283)
  line L6882 (130.441, -91.5876) -> (130.345, -91.7119)
  line L6883 (130.345, -91.7119) -> (130.221, -91.8072)
  line L6884 (129.497, -90.8633) -> (129.621, -90.768)
  line L6885 (135.802, -71.2333) -> (135.943, -71.3229)
  line L6886 (130.501, -91.1323) -> (130.521, -91.2876)
  line L6887 (129.321, -91.2876) -> (129.341, -91.1323)
  line L6888 (129.921, -90.6876) -> (130.076, -90.708)
  line L6889 (129.766, -90.708) -> (129.921, -90.6876)
  line L6890 (129.621, -91.8072) -> (129.497, -91.7119)
  line L6891 (129.401, -90.9876) -> (129.497, -90.8633)
  line L6892 (136.223, -71.9283) -> (136.2, -72.0939)
  line L6893 (133.968, -83.4302) -> (133.974, -83.4603)
  line L6894 (133.983, -83.4898) -> (133.983, -90.5263)
  line L6895 (134.013, -90.5302) -> (134.158, -90.5902)
  line L6896 (133.974, -83.4603) -> (133.983, -83.4898)
  line L6897 (135.645, -71.1772) -> (135.802, -71.2333)
  line L6898 (134.158, -90.5902) -> (134.282, -90.6855)
  line L6899 (136.141, -72.2502) -> (136.048, -72.3895)
  line L6900 (130.501, -91.4429) -> (130.441, -91.5876)
  line L6901 (135.598, -81.6204) -> (135.595, -81.6424)
  line L6902 (130.076, -90.708) -> (130.221, -90.768)
  line L6903 (129.341, -91.1323) -> (129.401, -90.9876)
  line L6904 (130.221, -91.8072) -> (130.076, -91.8672)
  line L6905 (134.458, -91.1098) -> (134.438, -91.2651)
  line L6906 (135.595, -81.6424) -> (135.596, -81.647)
  line L6907 (134.282, -90.6855) -> (134.378, -90.8098)
  line L6908 (135.927, -72.5048) -> (135.783, -72.5904)
  line L6909 (135.593, -81.6559) -> (135.577, -81.6817)
  line L6910 (112.339, -92.1904) -> (112.364, -92.209)
  line L6911 (111.46, -92.5547) -> (111.52, -92.41)
  line L6912 (110.166, -94.4335) -> (110.167, -94.4271)
  line L6913 (111.739, -92.1904) -> (111.884, -92.1304)
  line L6914 (110.162, -95.7837) -> (110.162, -94.4626)
  line L6915 (110.184, -94.4012) -> (110.198, -94.3742)
  line L6916 (110.126, -95.7875) -> (110.162, -95.7837)
  line L6917 (112.364, -92.209) -> (113.348, -91.2246)
  line L6918 (113.436, -91.188) -> (124.282, -91.188)
  line L6919 (109.967, -95.8414) -> (110.126, -95.7875)
  line L6920 (110.165, -94.4406) -> (110.165, -94.436)
  line L6921 (111.884, -92.1304) -> (112.039, -92.11)
  line L6922 (113.377, -91.2031) -> (113.407, -91.1967)
  line L6923 (113.407, -91.1967) -> (113.436, -91.188)
  line L6924 (109.825, -95.929) -> (109.967, -95.8414)
  line L6925 (112.195, -92.1304) -> (112.339, -92.1904)
  line L6926 (113.366, -91.2113) -> (113.369, -91.2078)
  line L6927 (111.46, -92.8653) -> (111.439, -92.71)
  line L6928 (111.439, -92.71) -> (111.46, -92.5547)
  line L6929 (111.52, -93.01) -> (111.46, -92.8653)
  line L6930 (111.615, -92.2857) -> (111.739, -92.1904)
  line L6931 (110.198, -94.3742) -> (111.538, -93.0342)
  line L6932 (111.52, -92.41) -> (111.615, -92.2857)
  line L6933 (109.706, -96.046) -> (109.825, -95.929)
  line L6934 (113.369, -91.2078) -> (113.372, -91.207)
  line L6935 (111.538, -93.0342) -> (111.52, -93.01)
  line L6936 (110.165, -94.436) -> (110.166, -94.4335)
  line L6937 (110.162, -94.4626) -> (110.165, -94.4406)
  line L6938 (131.747, -96.9696) -> (131.347, -96.9696)
  line L6939 (132.355, -95.8354) -> (132.353, -95.8379)
  line L6940 (134.017, -96.8204) -> (134.002, -96.8969)
  line L6941 (132.353, -95.8379) -> (132.352, -95.8443)
  line L6942 (131.931, -96.8461) -> (131.888, -96.911)
  line L6943 (133.24, -96.1825) -> (133.276, -96.129)
  line L6944 (132.613, -94.9999) -> (132.556, -95.1114)
  line L6945 (132.556, -94.6412) -> (132.613, -94.7527)
  line L6946 (131.909, -95.1114) -> (131.852, -94.9999)
  line L6947 (133.817, -96.0704) -> (133.894, -96.0856)
  line L6948 (131.997, -95.1999) -> (131.909, -95.1114)
  line L6949 (132.556, -95.1114) -> (132.468, -95.1999)
  line L6950 (131.162, -96.1431) -> (131.205, -96.0782)
  line L6951 (131.888, -96.911) -> (131.823, -96.9544)
  line L6952 (133.276, -96.129) -> (133.341, -96.0856)
  line L6953 (134.017, -96.2704) -> (134.017, -96.8204)
  line L6954 (124.282, -91.188) -> (124.304, -91.1912)
  line L6955 (132.109, -94.4959) -> (132.232, -94.4763)
  line L6956 (131.852, -94.9999) -> (131.832, -94.8763)
  line L6957 (132.357, -95.2998) -> (133.24, -96.1825)
  line L6958 (134.002, -96.1939) -> (134.017, -96.2704)
  line L6959 (132.356, -94.4959) -> (132.468, -94.5527)
  line L6960 (131.205, -96.0782) -> (131.27, -96.0348)
  line L6961 (132.232, -94.4763) -> (132.356, -94.4959)
  line L6962 (133.959, -96.9618) -> (133.894, -97.0052)
  line L6963 (133.417, -97.0204) -> (133.341, -97.0052)
  line L6964 (131.27, -96.0348) -> (131.347, -96.0196)
  line L6965 (131.997, -94.5527) -> (132.109, -94.4959)
  line L6966 (131.347, -96.9696) -> (131.27, -96.9544)
  line L6967 (132.613, -94.7527) -> (132.632, -94.8763)
  line L6968 (133.341, -96.0856) -> (133.417, -96.0704)
  line L6969 (133.341, -97.0052) -> (133.276, -96.9618)
  line L6970 (133.276, -96.9618) -> (133.232, -96.8969)
  line L6971 (133.232, -96.8969) -> (133.217, -96.8204)
  line L6972 (134.002, -96.8969) -> (133.959, -96.9618)
  line L6973 (132.468, -94.5527) -> (132.556, -94.6412)
  line L6974 (131.147, -96.2196) -> (131.162, -96.1431)
  line L6975 (131.347, -96.0196) -> (131.747, -96.0196)
  line L6976 (131.852, -94.7527) -> (131.909, -94.6412)
  line L6977 (133.817, -97.0204) -> (133.417, -97.0204)
  line L6978 (133.959, -96.129) -> (134.002, -96.1939)
  line L6979 (131.162, -96.8461) -> (131.147, -96.7696)
  line L6980 (131.947, -96.2714) -> (131.947, -96.7696)
  line L6981 (131.909, -94.6412) -> (131.997, -94.5527)
  line L6982 (133.894, -97.0052) -> (133.817, -97.0204)
  line L6983 (132.632, -94.8763) -> (132.613, -94.9999)
  line L6984 (132.357, -95.256) -> (132.357, -95.2998)
  line L6985 (132.357, -95.8088) -> (132.354, -95.8308)
  line L6986 (132.354, -95.8308) -> (132.355, -95.8354)
  line L6987 (110.167, -94.4271) -> (110.184, -94.4012)
  line L6988 (131.832, -94.8763) -> (131.852, -94.7527)
  line L6989 (133.217, -96.8204) -> (133.217, -96.5132)
  line L6990 (132.352, -95.8443) -> (132.336, -95.8702)
  line L6991 (132.468, -95.1999) -> (132.357, -95.256)
  line L6992 (113.372, -91.207) -> (113.377, -91.2031)
  line L6993 (133.417, -96.0704) -> (133.817, -96.0704)
  line L6994 (131.27, -96.9544) -> (131.205, -96.911)
  line L6995 (132.321, -95.8972) -> (131.947, -96.2714)
  line L6996 (133.217, -96.5132) -> (132.357, -95.6534)
  line L6997 (131.823, -96.9544) -> (131.747, -96.9696)
  line L6998 (131.147, -96.7696) -> (131.147, -96.2196)
  line L6999 (132.357, -95.6534) -> (132.357, -95.8088)
  line L7000 (133.894, -96.0856) -> (133.959, -96.129)
  line L7001 (146.324, -71.7412) -> (146.343, -71.9074)
  line L7002 (141.628, -83.4313) -> (141.628, -91.6947)
  line L7003 (131.823, -96.0348) -> (131.827, -96.0374)
  line L7004 (132.336, -95.8702) -> (132.321, -95.8972)
  line L7005 (131.205, -96.911) -> (131.162, -96.8461)
  line L7006 (131.747, -96.0196) -> (131.823, -96.0348)
  line L7007 (141.659, -91.6986) -> (141.803, -91.7586)
  line L7008 (131.947, -96.7696) -> (131.931, -96.8461)
  line L7009 (145.715, -79.3168) -> (145.714, -79.3192)
  line L7010 (146.167, -72.3895) -> (146.046, -72.5048)
  line L7011 (132.107, -95.256) -> (131.997, -95.1999)
  line L7012 (145.903, -72.5904) -> (145.744, -72.6421)
  line L7013 (145.764, -71.1772) -> (145.922, -71.2333)
  line L7014 (145.718, -79.2901) -> (145.715, -79.3122)
  line L7015 (132.107, -95.757) -> (132.107, -95.256)
  line L7016 (146.046, -72.5048) -> (145.903, -72.5904)
  line L7017 (141.384, -83.344) -> (141.4, -83.3182)
  line L7018 (142.023, -92.5782) -> (142.004, -92.6024)
  line L7019 (142.744, -96.1939) -> (142.788, -96.129)
  line L7020 (143.239, -93.8442) -> (143.245, -93.8743)
  line L7021 (142.788, -96.9618) -> (142.744, -96.8969)
  line L7022 (143.231, -93.8332) -> (143.234, -93.8363)
  line L7023 (143.004, -93.9556) -> (141.828, -92.7792)
  line L7024 (145.715, -79.3122) -> (145.715, -79.3168)
  line L7025 (145.713, -79.3256) -> (145.696, -79.3515)
  line L7026 (146.063, -71.3229) -> (146.181, -71.4415)
  line L7027 (146.269, -71.5833) -> (146.324, -71.7412)
  line L7028 (141.628, -91.6947) -> (141.659, -91.6986)
  line L7029 (145.718, -72.6444) -> (145.718, -79.2901)
  line L7030 (143.406, -96.0856) -> (143.47, -96.129)
  line L7031 (143.514, -96.8969) -> (143.47, -96.9618)
  line L7032 (143.217, -93.8154) -> (143.231, -93.8332)
  line L7033 (143.234, -93.8363) -> (143.235, -93.839)
  line L7034 (143.329, -97.0204) -> (142.929, -97.0204)
  line L7035 (143.529, -96.8204) -> (143.514, -96.8969)
  line L7036 (142.729, -96.8204) -> (142.729, -96.2704)
  line L7037 (141.928, -91.8539) -> (142.023, -91.9782)
  line L7038 (145.922, -71.2333) -> (146.063, -71.3229)
  line L7039 (142.729, -96.2704) -> (142.744, -96.1939)
  line L7040 (141.803, -91.7586) -> (141.928, -91.8539)
  line L7041 (146.343, -71.9074) -> (146.343, -71.9283)
  line L7042 (142.788, -96.129) -> (142.852, -96.0856)
  line L7043 (143.235, -93.839) -> (143.239, -93.8442)
  line L7044 (146.26, -72.2502) -> (146.167, -72.3895)
  line L7045 (142.083, -92.1229) -> (142.103, -92.2782)
  line L7046 (142.004, -92.6024) -> (143.217, -93.8154)
  line L7047 (146.343, -71.9283) -> (146.319, -72.0939)
  line L7048 (142.083, -92.4335) -> (142.023, -92.5782)
  line L7049 (143.47, -96.9618) -> (143.406, -97.0052)
  line L7050 (143.245, -93.8743) -> (143.254, -93.9038)
  line L7051 (143.514, -96.1939) -> (143.529, -96.2704)
  line L7052 (142.103, -92.2782) -> (142.083, -92.4335)
  line L7053 (142.023, -91.9782) -> (142.083, -92.1229)
  line L7054 (143.47, -96.129) -> (143.514, -96.1939)
  line L7055 (143.254, -96.0704) -> (143.329, -96.0704)
  line L7056 (143.406, -97.0052) -> (143.329, -97.0204)
  line L7057 (145.714, -79.3192) -> (145.713, -79.3256)
  line L7058 (145.681, -79.3785) -> (141.628, -83.4313)
  line L7059 (145.744, -72.6421) -> (145.718, -72.6444)
  line L7060 (143.529, -96.2704) -> (143.529, -96.8204)
  line L7061 (146.319, -72.0939) -> (146.26, -72.2502)
  line L7062 (145.696, -79.3515) -> (145.681, -79.3785)
  line L7063 (143.329, -96.0704) -> (143.406, -96.0856)
  line L7064 (143.254, -93.9038) -> (143.254, -96.0704)
  line L7065 (146.181, -71.4415) -> (146.269, -71.5833)
  line L7066 (131.827, -96.0374) -> (132.107, -95.757)
  line L7067 (142.929, -97.0204) -> (142.852, -97.0052)
  line L7068 (142.744, -96.8969) -> (142.729, -96.8204)
  line L7069 (142.852, -97.0052) -> (142.788, -96.9618)
  line L7070 (141.378, -83.3795) -> (141.382, -83.3575)
  line L7071 (111.581, -88.6411) -> (111.578, -88.6398)
  line L7072 (112.957, -87.9394) -> (113.101, -87.9994)
  line L7073 (141.383, -83.3504) -> (141.384, -83.344)
  line L7074 (145.273, -71.2288) -> (145.432, -71.1749)
  line L7075 (144.912, -72.222) -> (144.859, -72.0633)
  line L7076 (144.843, -71.8969) -> (144.864, -71.731)
  line L7077 (141.203, -92.7978) -> (141.079, -92.7025)
  line L7078 (141.079, -91.8539) -> (141.203, -91.7586)
  line L7079 (141.382, -83.3575) -> (141.381, -83.3529)
  line L7080 (142.929, -96.0704) -> (143.004, -96.0704)
  line L7081 (143.004, -96.0704) -> (143.004, -93.9556)
  line L7082 (140.984, -91.9782) -> (141.079, -91.8539)
  line L7083 (144.999, -72.365) -> (144.912, -72.222)
  line L7084 (145.115, -72.4853) -> (144.999, -72.365)
  line L7085 (141.381, -83.3529) -> (141.383, -83.3504)
  line L7086 (141.348, -92.8578) -> (141.203, -92.7978)
  line L7087 (141.503, -92.8782) -> (141.348, -92.8578)
  line L7088 (140.924, -92.1229) -> (140.984, -91.9782)
  line L7089 (141.203, -91.7586) -> (141.348, -91.6986)
  line L7090 (140.924, -92.4335) -> (140.903, -92.2782)
  line L7091 (145.468, -79.2384) -> (145.468, -72.6427)
  line L7092 (113.381, -88.6743) -> (113.321, -88.819)
  line L7093 (144.921, -71.5739) -> (145.012, -71.4334)
  line L7094 (141.4, -83.3182) -> (141.415, -83.2912)
  line L7095 (141.659, -92.8578) -> (141.503, -92.8782)
  line L7096 (145.012, -71.4334) -> (145.131, -71.3164)
  line L7097 (112.801, -89.119) -> (112.646, -89.0986)
  line L7098 (112.218, -88.644) -> (111.608, -88.644)
  line L7099 (112.222, -88.6743) -> (112.218, -88.644)
  line L7100 (141.415, -83.2912) -> (145.468, -79.2384)
  line L7101 (145.468, -72.6427) -> (145.411, -72.6351)
  line L7102 (144.864, -71.731) -> (144.921, -71.5739)
  line L7103 (141.378, -91.6947) -> (141.378, -83.3795)
  line L7104 (113.226, -88.9433) -> (113.101, -89.0386)
  line L7105 (141.079, -92.7025) -> (140.984, -92.5782)
  line L7106 (113.321, -88.219) -> (113.381, -88.3637)
  line L7107 (113.381, -88.3637) -> (113.401, -88.519)
  line L7108 (140.903, -92.2782) -> (140.924, -92.1229)
  line L7109 (113.101, -87.9994) -> (113.226, -88.0947)
  line L7110 (145.255, -72.5768) -> (145.115, -72.4853)
  line L7111 (140.984, -92.5782) -> (140.924, -92.4335)
  line L7112 (112.282, -88.819) -> (112.222, -88.6743)
  line L7113 (111.586, -88.6408) -> (111.581, -88.6411)
  line L7114 (141.348, -91.6986) -> (141.378, -91.6947)
  line L7115 (113.321, -88.819) -> (113.226, -88.9433)
  line L7116 (113.401, -88.519) -> (113.381, -88.6743)
  line L7117 (145.411, -72.6351) -> (145.255, -72.5768)
  line L7118 (141.803, -92.7978) -> (141.659, -92.8578)
  line L7119 (145.131, -71.3164) -> (145.273, -71.2288)
  line L7120 (112.646, -89.0986) -> (112.501, -89.0386)
  line L7121 (113.226, -88.0947) -> (113.321, -88.219)
  line L7122 (141.828, -92.7792) -> (141.803, -92.7978)
  line L7123 (144.859, -72.0633) -> (144.843, -71.8969)
  line L7124 (142.852, -96.0856) -> (142.929, -96.0704)
  line L7125 (111.608, -88.644) -> (111.586, -88.6408)
  line L7126 (95.0022, -90.5981) -> (95.0031, -90.5917)
  line L7127 (94.998, -95.1474) -> (94.998, -90.6272)
  line L7128 (94.711, -95.7835) -> (94.7079, -95.787)
  line L7129 (95.2261, -95.2606) -> (95.2114, -95.2876)
  line L7130 (145.598, -71.1574) -> (145.764, -71.1772)
  line L7131 (92.227, -95.7771) -> (91.7488, -95.7653)
  line L7132 (97.3714, -88.202) -> (97.3892, -88.1887)
  line L7133 (91.1387, -95.3074) -> (91.2502, -95.2506)
  line L7134 (91.609, -95.9546) -> (91.4975, -96.0114)
  line L7135 (91.3739, -95.231) -> (91.4975, -95.2506)
  line L7136 (94.7052, -95.7878) -> (94.7, -95.7917)
  line L7137 (90.9597, -95.6472) -> (90.9797, -95.5939)
  line L7138 (113.101, -89.0386) -> (112.957, -89.0986)
  line L7139 (94.7288, -95.7702) -> (94.711, -95.7835)
  line L7140 (90.9908, -95.7378) -> (90.9745, -95.716)
  line L7141 (95.2448, -95.2212) -> (95.2451, -95.2258)
  line L7142 (94.6699, -95.7981) -> (94.6404, -95.8068)
  line L7143 (91.1387, -95.9546) -> (91.0502, -95.8661)